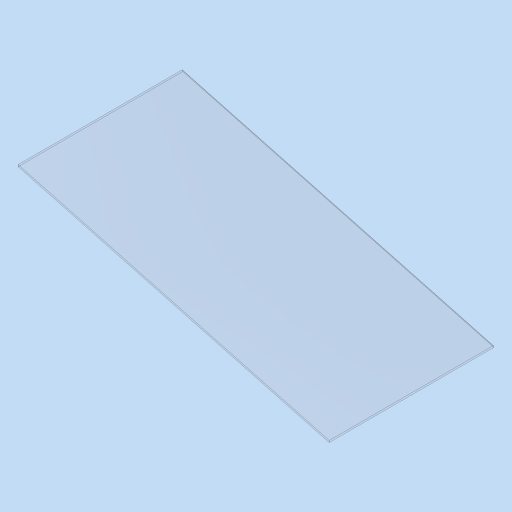
# Autodesk Inventor part: 부품2
Saved by Autodesk Inventor 2024 (Build 280153000, 153)
## iProperties
Created: 2024-01-19
Part Number: 부품2
Material: 에폭시 수지
Document SubType Name: Modeling
Designer: KBU
Density: 1.14 g/cm^3
Appearance: 투명 - 슬레이트 파란색
Author: KBU
Autodesk Inventor part; units mm, degrees
ref_plane "YZ Plane" through (0, 0, 0) normal (1, 0, 0) x (0, 1, 0)
ref_plane "XZ Plane" through (0, 0, 0) normal (0, 1, 0) x (-1, 0, 0)
ref_plane "XY Plane" through (0, 0, 0) normal (0, 0, 1) x (1, 0, 0)
sketch "스케치1" plane through (0, 0, 0) normal (0, 0, 1) x (1, 0, 0)
  line L0 (0, 0) -> (0, 5)
  line L1 (0, 0) -> (-850, 227.7568)
  line L2 (-12.9463, 0) -> (8.7754, 0)
  line L3 (0, 5) -> (-850, 232.7568)
  line L4 (-850, 227.7568) -> (-850, 232.7568)
  point P0 (-850, 230.2568)
  point P1 (-850, 242.7568)
  point P2 (0, 15)
  dimension "d0" = 15
  dimension "d1" = 5
  dimension "d2" = 850
  constraints: 10 end point, 2 point on line, 2 vertical, 1 coincident, 1 horizontal, 1 midpoint, 1 parallel
  measures "d0" angle of L1 L2
  measures "d1" distance of L0.start L0.end
  measures "d2" distance from line of L0 point (-850, 230.257)
extrude "돌출1" add sketch "스케치1" against normal blind 450
sketch "스케치3" plane through (0, 15, 0) normal (0.2588, 0.9659, 0) x (0.9659, -0.2588, 0)
  line L0 (-879.9848, 0) -> (-879.9848, 450) projected
  line L1 (3.8823, 0) -> (3.8823, 450) projected
  spline S0 degree 4 poles (-879.9848, 225) (-790.3669, 315.2357) (-705.7025, 105.8229) (-615.8925, 383.2001) (-422.1913, 176.8706) (-352.8385, 360.4529) (-185.1098, 145.8092) (-106.461, 355.2219) (-47.5696, 282.9867) (3.8823, 225) knots 0 0 0 0 0 0.288179 0.401252 0.519809 0.635267 0.741109 1 1 1 1 1
  line L2 (-879.9848, 225) -> (-986.5845, 327.8412)
  line L3 (-986.5845, 327.8412) -> (-911.355, 729.5985)
  line L4 (-911.355, 729.5985) -> (113.0461, 683.1803)
  line L5 (113.0461, 683.1803) -> (3.8823, 225)
  point P0 (-751.2924, 234.868)
  point P1 (-666.4591, 234.868)
  point P2 (-560.8178, 275.0205)
  point P3 (-432.7676, 244.6086)
  point P4 (-339.9313, 291.6979)
  point P5 (-223.0855, 244.6086)
  point P6 (-138.2523, 275.0205)
  point P7 (-77.4285, 291.6979)
  constraints: 8 end point, 2 midpoint, 10 other
extrude "돌출3" [suppressed]
fillet "모깎기4" [suppressed]
fillet "모깎기5" radius 2 1 edges at (-425, 118.8784, -450)
